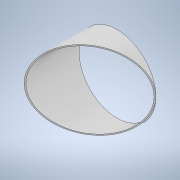
# Autodesk Inventor part: SolarPanel
Saved by Autodesk Inventor 2021 (Build 250183000, 183)
## iProperties
Created: 2021-03-06
Part Number: SolarPanel
Material: Generic
Document SubType Name: Modeling
Designer: allen
Density: 1 g/cm^3
Appearance: Default
Author: allen
Autodesk Inventor part; units mm, degrees
ref_plane "YZ Plane" through (0, 0, 0) normal (1, 0, 0) x (0, 1, 0)
ref_plane "XZ Plane" through (0, 0, 0) normal (0, 1, 0) x (-1, 0, 0)
ref_plane "XY Plane" through (0, 0, 0) normal (0, 0, 1) x (1, 0, 0)
sketch "Sketch1" plane through (0, 0, 0) normal (0, 0, 1) x (1, 0, 0)
  circle A0 centre (0, 0) radius 70
  circle A1 centre (0, 0) radius 72
  dimension "d0" = 140
  dimension "d1" = 144
  constraints: 2 centre point, 2 coincident
  measures "d0" diameter of A0
  measures "d1" diameter of A1
sketch "Sketch3" plane through (0, 0, 0) normal (0, 1, 0) x (-1, 0, 0)
  line L0 (-72, 0) -> (-72, 200)
  line L1 (-72, 200) -> (216, 200)
  line L2 (216, 200) -> (-72, 0)
  point P0 (0, 0)
  dimension "d2" = 288
  dimension "d3" = 72
  dimension "d4" = 200
  dimension "d5" = 200
  constraints: 6 end point, 1 perpendicular, 1 vertical
  measures "d2" distance of L0.end L1.end
  measures "d3" distance from line of L0 point (0, 0)
  measures "d4" distance of L0.start L0.end
  measures "d5" distance from line of point (0, 0) L1
extrude "Extrusion1" add sketch "Sketch1" along normal blind 100
extrude "Extrusion2" cut sketch "Sketch3" along normal mid plane 200
body "Solid1"
